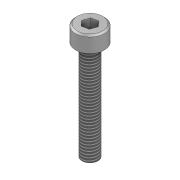
# Autodesk Inventor part: Tornillo Allen cabeza cilindrica M4x25mm
Saved by Autodesk Inventor 2020.3 (Build 243373000, 373)
## iProperties
Created: 2020-05-08
Part Number: Tornillo Allen cabeza cilindrica M4x25mm
Material: Generic
Document SubType Name: Modeling
Designer: Dante
Density: 1 g/cm^3
Appearance: Goma - Negro - Versión 1.1
Author: Dante
Autodesk Inventor part; units mm, degrees
ref_plane "YZ Plane" through (0, 0, 0) normal (1, 0, 0) x (0, 1, 0)
ref_plane "XZ Plane" through (0, 0, 0) normal (0, 1, 0) x (-1, 0, 0)
ref_plane "XY Plane" through (0, 0, 0) normal (0, 0, 1) x (1, 0, 0)
sketch "Sketch1" plane through (0, 0, 0) normal (0, 0, 1) x (1, 0, 0)
  line L0 (-9.9228, -30) -> (-13.5328, -30)
  line L1 (-13.5328, -30) -> (-13.5328, -26)
  line L2 (-13.5328, -26) -> (-9.9228, -26)
  line L3 (-9.9228, -26) -> (-9.9228, -30)
  line L4 (-9.9228, -30) -> (-9.9228, -55)
  line L5 (-9.9228, -55) -> (-11.9228, -55)
  line L6 (-11.9228, -55) -> (-11.9228, -30)
  point P0 (0, 0)
  dimension "d0" = 3.61
  dimension "d1" = 4
  dimension "d3" = 2
  dimension "d16" = 25
  constraints: 14 end point, 4 perpendicular, 2 vertical, 1 horizontal, 1 point on line
  measures "d0" distance of L0.start L0.end
  measures "d1" distance of L0.end L1.end
  measures "d3" distance of L4.end L5.end
  measures "d16" distance from line of L4.end L0
revolve "Revolution1" add sketch "Sketch1" angle 360 about axis through (-9.9228, -30, 0) along (0, -1, 0)
chamfer "Chamfer1" distance 0.4 angle 45 1 edges at (-6.3128, -26, 0)
sketch "Boceto2" plane through (-9.9228, -26, 0) normal (0, 1, 0) x (1, 0, 0)
  line L0 (1.1641, -1.3443) -> (-0.5821, -1.6803)
  line L1 (-0.5821, -1.6803) -> (-1.7462, -0.336)
  line L2 (-1.7462, -0.336) -> (-1.1641, 1.3443)
  line L3 (-1.1641, 1.3443) -> (0.5821, 1.6803)
  line L4 (0.5821, 1.6803) -> (1.7462, 0.336)
  line L5 (1.7462, 0.336) -> (1.1641, -1.3443)
  point P0 (9.9228, 0)
  point P1 (0, 0)
  dimension "d11" = 3.08
  constraints: 12 end point, 13 other
  measures "d11" distance between parallel lines of L5 L2
extrude "Extrusión1" cut sketch "Boceto2" against normal blind 2
thread "Rosca1" size "M4x0.7" class "6g" standard "ISO Metric profile" length 430
body "Solid1"
